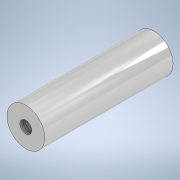
# Autodesk Inventor part: Barras_Soporte_superior
Saved by Autodesk Inventor 2021 (Build 250183000, 183)
## iProperties
Created: 2021-04-19
Part Number: Barras_Soporte_superior
Material: Acero inoxidable
Document SubType Name: Modeling
Designer: Admin
Density: 8 g/cm^3
Appearance: Aluminio - Oscuro
Author: Admin
Autodesk Inventor part; units mm, degrees
ref_plane "YZ Plane" through (0, 0, 0) normal (1, 0, 0) x (0, 1, 0)
ref_plane "XZ Plane" through (0, 0, 0) normal (0, 1, 0) x (-1, 0, 0)
ref_plane "XY Plane" through (0, 0, 0) normal (0, 0, 1) x (1, 0, 0)
sketch "Boceto1" plane through (0, 0, 0) normal (0, 0, 1) x (1, 0, 0)
  circle A0 centre (0, 0) radius 7.94
  dimension "d0" = 15.88
  constraints: 1 centre point, 1 coincident
  measures "d0" diameter of A0
extrude "Extrusión1" add sketch "Boceto1" along normal blind 53.74
sketch "Boceto4" plane through (0, 0, 0) normal (0, 0, -1) x (-1, 0, 0)
  circle A0 centre (0, 0) radius 1.7349
  constraints: 1 centre point, 1 coincident
sketch "Boceto5" plane through (0, 0, 53.74) normal (0, 0, 1) x (1, 0, 0)
  circle A0 centre (0, 0) radius 2.5
  dimension "d17" = 5
  constraints: 1 centre point, 1 coincident
  measures "d17" diameter of A0
hole "Agujero1" at (0, 0, 0) direction (0, 0, 1) diameter 5 depth 10 tip angle 118
hole "Agujero2" at (0, 0, 53.74) direction (0, 0, -1) diameter 5 depth 10 tip angle 118
thread "Rosca5" size "M5x0.8" class "6H" standard "ANSI Metric M Profile" length 8
thread "Rosca6" size "M5x0.8" class "6H" standard "ANSI Metric M Profile" length 8
